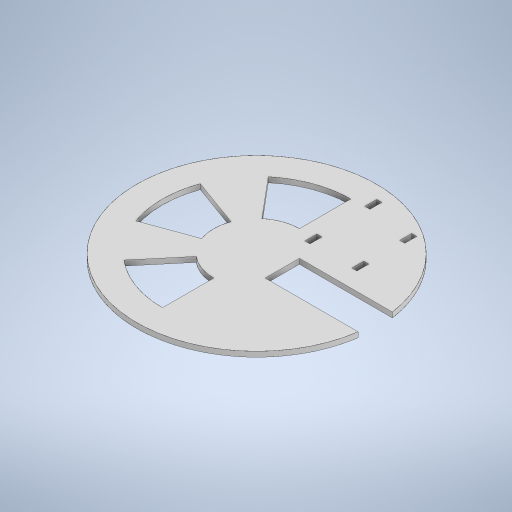
# Autodesk Inventor part: rolling_plate_top
Saved by Autodesk Inventor 2024 (Build 280153000, 153)
## iProperties
Created: 2024-04-09
Part Number: rolling_plate_top
Material: 一般
Document SubType Name: Modeling
Designer: USER
Density: 1 g/cm^3
Appearance: 預設
Author: USER
Autodesk Inventor part; units mm, degrees
ref_plane "YZ Plane" through (0, 0, 0) normal (1, 0, 0) x (0, 1, 0)
ref_plane "XZ Plane" through (0, 0, 0) normal (0, 1, 0) x (-1, 0, 0)
ref_plane "XY Plane" through (0, 0, 0) normal (0, 0, 1) x (1, 0, 0)
sketch "草圖1" plane through (0, 0, 0) normal (0, 1, 0) x (-1, 0, 0)
  circle A0 centre (0, 0) radius 70
  circle A1 centre (0, 0) radius 25
  line L0 (-70, 10) -> (-15, 10)
  line L1 (-15, 10) -> (-15, -10)
  line L2 (-15, -10) -> (-70, -10)
  line L3 (-70, -10) -> (-70, 10)
  line L4 (0, 0) -> (0, -55)
  line L5 (0, 0) -> (35.3533, -42.1324)
  arc A2 (0, -55) -> (35.3533, -42.1324) centre (0, 0) ccw
  line L6 (0, 0) -> (51.6831, -18.8111)
  line L7 (0, 0) -> (51.6831, 18.8111)
  arc A3 (51.6831, -18.8111) -> (51.6831, 18.8111) centre (0, 0) ccw
  line L8 (0, 0) -> (35.3533, 42.1324)
  line L9 (0, 0) -> (0, 55)
  arc A4 (35.3533, 42.1324) -> (0, 55) centre (0, 0) ccw
  line L10 (-9.3, -13.3795) -> (-36.7, -13.3795)
  line L11 (-36.7, -13.3795) -> (-36.7, -69.3795)
  line L12 (-36.7, -69.3795) -> (-9.3, -69.3795)
  line L13 (-9.3, -69.3795) -> (-9.3, -13.3795)
  line L14 (-7.8, -20.3795) -> (-10.8, -20.3795)
  line L15 (-10.8, -20.3795) -> (-10.8, -27.3795)
  line L16 (-10.8, -27.3795) -> (-7.8, -27.3795)
  line L17 (-7.8, -27.3795) -> (-7.8, -20.3795)
  line L18 (-7.8, -55.3795) -> (-10.8, -55.3795)
  line L19 (-10.8, -55.3795) -> (-10.8, -62.3795)
  line L20 (-10.8, -62.3795) -> (-7.8, -62.3795)
  line L21 (-7.8, -62.3795) -> (-7.8, -55.3795)
  line L22 (-35.2, -20.3795) -> (-38.2, -20.3795)
  line L23 (-38.2, -20.3795) -> (-38.2, -27.3795)
  line L24 (-38.2, -27.3795) -> (-35.2, -27.3795)
  line L25 (-35.2, -27.3795) -> (-35.2, -20.3795)
  line L26 (-35.2, -48.3795) -> (-38.2, -48.3795)
  line L27 (-38.2, -48.3795) -> (-38.2, -55.3795)
  line L28 (-38.2, -55.3795) -> (-35.2, -55.3795)
  line L29 (-35.2, -55.3795) -> (-35.2, -48.3795)
  circle A5 centre (0, 0) radius 2
  line L30 (-1.5, 1.3229) -> (-1.5, -1.3229)
  point P0 (-23, -13.3795)
  point P1 (-9.3, -20.3795)
  point P2 (-9.3, -62.3795)
  point P3 (-36.7, -20.3795)
  point P4 (-36.7, -48.3795)
  point P5 (16.0697, -19.1511)
  point P6 (0, -25)
  point P7 (-69.282, 10)
  point P8 (-69.282, -10)
  point P9 (16.0697, 19.1511)
  point P10 (0, 25)
  point P11 (23.4923, -8.5505)
  point P12 (23.4923, 8.5505)
  point P13 (-70, 0)
  dimension "d0" = 140
  dimension "d1" = 50
  dimension "d2" = 20
  dimension "d3" = 55
  dimension "d4" = 55
  dimension "d5" = 40
  dimension "d6" = 55
  dimension "d9" = 140
  dimension "d11" = 8
  dimension "d12" = 27.4
  dimension "d13" = 56
  dimension "d14" = 7
  dimension "d15" = 3
  dimension "d16" = 7
  dimension "d17" = 7
  dimension "d18" = 3
  dimension "d19" = 7
  dimension "d20" = 7
  dimension "d21" = 3
  dimension "d22" = 7
  dimension "d23" = 7
  dimension "d24" = 3
  dimension "d25" = 21
  dimension "d28" = 4
  dimension "d29" = 1.5
  constraints: 62 end point, 12 parallel, 10 point on circle, 6 centre point, 6 coincident, 6 horizontal, 6 midpoint, 6 perpendicular, 6 point on line, 2 vertical, 1 horizontal alignment, 1 vertical alignment, 17 other
  measures "d0" diameter of A0
  measures "d1" diameter of A1
  measures "d2" distance of L2.end L0.start
  measures "d3" distance of L1.end L2.end
  measures "d4" distance of L4.start L4.end
  measures "d5" angle of L4 L5
  measures "d6" distance of L4.start L5.end
  measures "d11" horizontal distance of L1.end point (-23, -13.379)
  measures "d12" distance of L11.end L12.end
  measures "d13" distance of L12.end L10.start
  measures "d14" distance of L16.end L14.start
  measures "d15" distance of L15.end L16.end
  measures "d16" distance from line of L10.start L14
  measures "d17" distance of L20.end L18.start
  measures "d18" distance of L19.end L20.end
  measures "d19" distance from line of L12.end L20
  measures "d20" distance of L24.end L22.start
  measures "d21" distance of L23.end L24.end
  measures "d22" vertical distance of L10.end L22.start
  measures "d23" distance of L28.end L26.start
  measures "d24" distance of L27.end L28.end
  measures "d25" distance of L24.end L26.start
  measures "d28" diameter of A5
  measures "d29" distance between parallel lines of L4 L30
extrude "擠出1" add sketch "草圖1" along normal blind 3 contours L13 L20 L21 L18 L16 L17 A1 L4 A2 L5 L6 A3 L7 L8 A4 L9 L0 A0 | A0 L11 L28 L29 L26 L24 L25 L22 L10 A1 L15 L16 L13 L18 L19 L20 | A0 L2 A1 L10 L11 L22 L23 L24 L26 L27 L28 | A1 L9 A5 L4 L17 L14 L13 L10 L2 L1 L0 | A1 L8 A5 L9 | L10 L13 L14 L15 A1 | A1 L7 A5 L8 | A5 L8 L9 | L9 L4 A5 L30 | A1 L6 A5 L7 | A5 L7 L8 | L5 A5 L4 | L6 A5 L5 | L7 A5 L6 | L30 A5 | L4 A5 L5 A1 | A5 L6 A1 L5
